Autodesk Fusion 360 part; units mm, degrees
(part 2 of 4)
sketch "Sketch2 (2)" plane through (0, 0, 6) normal (0, 0, 1) x (-1, 0, 0)
  arc A0 (-38.0356, 4.8944) -> (-38.1711, 3.692) centre (0, 0) ccw
  arc A1 (-39.2367, 2.7907) -> (-38.1711, 3.692) centre (-39.1664, 3.7883) ccw
  line L0 (-39.2367, 2.7907) -> (-39.3676, 2.8)
  spline S0 degree 5 poles (-39.3676, 2.8) (-39.3839, 2.8011) (-39.4163, 2.803) (-39.4649, 2.8047) (-39.5299, 2.8047) (-39.6111, 2.8017) (-39.6923, 2.7966) (-39.7736, 2.79) (-39.855, 2.7828) (-39.9363, 2.775) (-40.0176, 2.7667) (-40.099, 2.7577) (-40.1803, 2.7478) (-40.2616, 2.7369) (-40.343, 2.7249) (-40.4243, 2.7119) (-40.5056, 2.6981) (-40.5868, 2.6836) (-40.6681, 2.6685) (-40.7493, 2.6528) (-40.8305, 2.6365) (-40.9117, 2.6196) (-40.9928, 2.6021) (-41.074, 2.5839) (-41.1551, 2.5651) (-41.2361, 2.5457) (-41.3171, 2.5256) (-41.3981, 2.505) (-41.4791, 2.4839) (-41.56, 2.4622) (-41.6408, 2.44) (-41.7216, 2.4173) (-41.8024, 2.3941) (-41.8832, 2.3703) (-41.9638, 2.346) (-42.0445, 2.3213) (-42.1251, 2.296) (-42.2056, 2.2702) (-42.2861, 2.244) (-42.3666, 2.2173) (-42.447, 2.1901) (-42.5273, 2.1624) (-42.6076, 2.1343) (-42.6878, 2.1058) (-42.768, 2.0768) (-42.8481, 2.0473) (-42.9282, 2.0174) (-43.0082, 1.9871) (-43.0881, 1.9563) (-43.168, 1.9251) (-43.2479, 1.8935) (-43.3276, 1.8614) (-43.4073, 1.829) (-43.4869, 1.7961) (-43.5665, 1.7628) (-43.646, 1.7291) (-43.7254, 1.695) (-43.8048, 1.6605) (-43.8841, 1.6256) (-43.9633, 1.5903) (-44.0425, 1.5546) (-44.1216, 1.5185) (-44.2006, 1.482) (-44.2795, 1.4452) (-44.3584, 1.4079) (-44.4372, 1.3703) (-44.5159, 1.3323) (-44.5946, 1.2939) (-44.6732, 1.2552) (-44.7516, 1.2161) (-44.8301, 1.1766) (-44.8927, 1.1447) (-44.9397, 1.1206) (-44.971, 1.1045) (-44.9866, 1.0964) knots 0 0 0 0 0 0 0.01428571 0.02857143 0.04285714 0.05714286 0.07142857 0.08571429 0.1 0.11428571 0.12857143 0.14285714 0.15714286 0.17142857 0.18571429 0.2 0.21428571 0.22857143 0.24285714 0.25714286 0.27142857 0.28571429 0.3 0.31428571 0.32857143 0.34285714 0.35714286 0.37142857 0.38571429 0.4 0.41428571 0.42857143 0.44285714 0.45714286 0.47142857 0.48571429 0.5 0.51428571 0.52857143 0.54285714 0.55714286 0.57142857 0.58571429 0.6 0.61428571 0.62857143 0.64285714 0.65714286 0.67142857 0.68571429 0.7 0.71428571 0.72857143 0.74285714 0.75714286 0.77142857 0.78571429 0.8 0.81428571 0.82857143 0.84285714 0.85714286 0.87142857 0.88571429 0.9 0.91428571 0.92857143 0.94285714 0.95714286 0.97142857 0.98571429 1 1 1 1 1 1
  arc A2 (-44.9866, 1.0964) -> (-44.9866, -1.0964) centre (0, 0) ccw
  spline S1 degree 5 poles (-44.9866, -1.0964) (-44.971, -1.1045) (-44.9397, -1.1206) (-44.8927, -1.1447) (-44.8301, -1.1766) (-44.7516, -1.2161) (-44.6732, -1.2552) (-44.5946, -1.2939) (-44.5159, -1.3323) (-44.4372, -1.3703) (-44.3584, -1.4079) (-44.2795, -1.4452) (-44.2006, -1.482) (-44.1216, -1.5185) (-44.0425, -1.5546) (-43.9633, -1.5903) (-43.8841, -1.6256) (-43.8048, -1.6605) (-43.7254, -1.695) (-43.646, -1.7291) (-43.5665, -1.7628) (-43.4869, -1.7961) (-43.4073, -1.829) (-43.3276, -1.8614) (-43.2479, -1.8935) (-43.168, -1.9251) (-43.0881, -1.9563) (-43.0082, -1.9871) (-42.9282, -2.0174) (-42.8481, -2.0473) (-42.768, -2.0768) (-42.6878, -2.1058) (-42.6076, -2.1343) (-42.5273, -2.1624) (-42.447, -2.1901) (-42.3666, -2.2173) (-42.2861, -2.244) (-42.2056, -2.2702) (-42.1251, -2.296) (-42.0445, -2.3213) (-41.9638, -2.346) (-41.8832, -2.3703) (-41.8024, -2.3941) (-41.7216, -2.4173) (-41.6408, -2.44) (-41.56, -2.4622) (-41.4791, -2.4839) (-41.3981, -2.505) (-41.3171, -2.5256) (-41.2361, -2.5457) (-41.1551, -2.5651) (-41.074, -2.5839) (-40.9928, -2.6021) (-40.9117, -2.6196) (-40.8305, -2.6365) (-40.7493, -2.6528) (-40.6681, -2.6685) (-40.5868, -2.6836) (-40.5056, -2.6981) (-40.4243, -2.7119) (-40.343, -2.7249) (-40.2616, -2.7369) (-40.1803, -2.7478) (-40.099, -2.7577) (-40.0176, -2.7667) (-39.9363, -2.775) (-39.855, -2.7828) (-39.7736, -2.79) (-39.6923, -2.7966) (-39.6111, -2.8017) (-39.5299, -2.8047) (-39.4649, -2.8047) (-39.4163, -2.803) (-39.3839, -2.8011) (-39.3676, -2.8) knots -1 -1 -1 -1 -1 -1 -0.98571429 -0.97142857 -0.95714286 -0.94285714 -0.92857143 -0.91428571 -0.9 -0.88571429 -0.87142857 -0.85714286 -0.84285714 -0.82857143 -0.81428571 -0.8 -0.78571429 -0.77142857 -0.75714286 -0.74285714 -0.72857143 -0.71428571 -0.7 -0.68571429 -0.67142857 -0.65714286 -0.64285714 -0.62857143 -0.61428571 -0.6 -0.58571429 -0.57142857 -0.55714286 -0.54285714 -0.52857143 -0.51428571 -0.5 -0.48571429 -0.47142857 -0.45714286 -0.44285714 -0.42857143 -0.41428571 -0.4 -0.38571429 -0.37142857 -0.35714286 -0.34285714 -0.32857143 -0.31428571 -0.3 -0.28571429 -0.27142857 -0.25714286 -0.24285714 -0.22857143 -0.21428571 -0.2 -0.18571429 -0.17142857 -0.15714286 -0.14285714 -0.12857143 -0.11428571 -0.1 -0.08571429 -0.07142857 -0.05714286 -0.04285714 -0.02857143 -0.01428571 0 0 0 0 0 0
  line L1 (-39.3676, -2.8) -> (-39.2367, -2.7907)
  arc A3 (-38.1711, -3.692) -> (-39.2367, -2.7907) centre (-39.1664, -3.7883) ccw
  arc A4 (-38.1711, -3.692) -> (-38.0356, -4.8944) centre (0, 0) ccw
  arc A5 (-38.874, -6.0102) -> (-38.0356, -4.8944) centre (-39.0274, -5.0221) ccw
  line L2 (-38.874, -6.0102) -> (-39.0037, -6.0303)
  spline S2 degree 5 poles (-39.0037, -6.0303) (-39.0197, -6.0328) (-39.0518, -6.0382) (-39.0996, -6.0474) (-39.1629, -6.0618) (-39.2414, -6.0828) (-39.3195, -6.1059) (-39.3973, -6.1304) (-39.4749, -6.1556) (-39.5525, -6.1813) (-39.63, -6.2074) (-39.7073, -6.2343) (-39.7844, -6.262) (-39.8612, -6.2908) (-39.9378, -6.3206) (-40.0142, -6.3513) (-40.0904, -6.3829) (-40.1664, -6.4151) (-40.2422, -6.4479) (-40.3179, -6.4813) (-40.3935, -6.5152) (-40.4689, -6.5498) (-40.5441, -6.5849) (-40.6191, -6.6207) (-40.694, -6.6571) (-40.7687, -6.6941) (-40.8432, -6.7316) (-40.9176, -6.7697) (-40.9918, -6.8084) (-41.0659, -6.8475) (-41.1398, -6.8871) (-41.2135, -6.9272) (-41.2871, -6.9679) (-41.3605, -7.009) (-41.4338, -7.0506) (-41.5069, -7.0927) (-41.5798, -7.1353) (-41.6526, -7.1783) (-41.7253, -7.2218) (-41.7978, -7.2658) (-41.8701, -7.3102) (-41.9423, -7.355) (-42.0143, -7.4003) (-42.0861, -7.4459) (-42.1579, -7.4921) (-42.2294, -7.5386) (-42.3008, -7.5856) (-42.3721, -7.633) (-42.4432, -7.6808) (-42.5141, -7.7289) (-42.5849, -7.7775) (-42.6555, -7.8265) (-42.726, -7.8759) (-42.7963, -7.9257) (-42.8665, -7.9759) (-42.9365, -8.0264) (-43.0063, -8.0773) (-43.076, -8.1286) (-43.1456, -8.1803) (-43.215, -8.2323) (-43.2842, -8.2848) (-43.3533, -8.3375) (-43.4222, -8.3907) (-43.491, -8.4442) (-43.5596, -8.498) (-43.628, -8.5523) (-43.6963, -8.6068) (-43.7644, -8.6617) (-43.8324, -8.717) (-43.9002, -8.7726) (-43.9679, -8.8285) (-44.0219, -8.8736) (-44.0623, -8.9075) (-44.0893, -8.9302) (-44.1027, -8.9415) knots 0 0 0 0 0 0 0.01428571 0.02857143 0.04285714 0.05714286 0.07142857 0.08571429 0.1 0.11428571 0.12857143 0.14285714 0.15714286 0.17142857 0.18571429 0.2 0.21428571 0.22857143 0.24285714 0.25714286 0.27142857 0.28571429 0.3 0.31428571 0.32857143 0.34285714 0.35714286 0.37142857 0.38571429 0.4 0.41428571 0.42857143 0.44285714 0.45714286 0.47142857 0.48571429 0.5 0.51428571 0.52857143 0.54285714 0.55714286 0.57142857 0.58571429 0.6 0.61428571 0.62857143 0.64285714 0.65714286 0.67142857 0.68571429 0.7 0.71428571 0.72857143 0.74285714 0.75714286 0.77142857 0.78571429 0.8 0.81428571 0.82857143 0.84285714 0.85714286 0.87142857 0.88571429 0.9 0.91428571 0.92857143 0.94285714 0.95714286 0.97142857 0.98571429 1 1 1 1 1 1
  arc A6 (-44.1027, -8.9415) -> (-43.6148, -11.0794) centre (0, 0) ccw
  spline S3 degree 5 poles (-43.6148, -11.0794) (-43.5977, -11.0838) (-43.5636, -11.0926) (-43.5125, -11.1056) (-43.4443, -11.1227) (-43.359, -11.1438) (-43.2738, -11.1644) (-43.1886, -11.1847) (-43.1034, -11.2046) (-43.0182, -11.2242) (-42.933, -11.2433) (-42.8478, -11.2621) (-42.7626, -11.2804) (-42.6775, -11.2984) (-42.5923, -11.316) (-42.5072, -11.3332) (-42.4221, -11.35) (-42.337, -11.3664) (-42.252, -11.3823) (-42.167, -11.3979) (-42.0819, -11.4131) (-41.997, -11.4278) (-41.912, -11.4422) (-41.8271, -11.4561) (-41.7422, -11.4696) (-41.6573, -11.4826) (-41.5725, -11.4953) (-41.4877, -11.5075) (-41.403, -11.5193) (-41.3183, -11.5306) (-41.2336, -11.5415) (-41.149, -11.5519) (-41.0644, -11.5619) (-40.9799, -11.5715) (-40.8954, -11.5805) (-40.811, -11.5891) (-40.7266, -11.5973) (-40.6423, -11.6049) (-40.558, -11.6121) (-40.4738, -11.6188) (-40.3897, -11.6251) (-40.3056, -11.6308) (-40.2216, -11.636) (-40.1377, -11.6406) (-40.0538, -11.6448) (-39.9701, -11.6484) (-39.8864, -11.6516) (-39.8028, -11.6542) (-39.7192, -11.6562) (-39.6358, -11.6577) (-39.5524, -11.6587) (-39.4692, -11.659) (-39.3861, -11.6586) (-39.303, -11.6577) (-39.2201, -11.656) (-39.1373, -11.6538) (-39.0547, -11.6511) (-38.9721, -11.6477) (-38.8896, -11.6438) (-38.8073, -11.6392) (-38.7251, -11.6337) (-38.6432, -11.6273) (-38.5615, -11.6199) (-38.48, -11.6114) (-38.3987, -11.6021) (-38.3175, -11.5921) (-38.2365, -11.5816) (-38.1556, -11.5706) (-38.0749, -11.5588) (-37.9945, -11.5458) (-37.9147, -11.5306) (-37.8514, -11.5162) (-37.8043, -11.5037) (-37.7731, -11.4946) (-37.7576, -11.4899) knots -1 -1 -1 -1 -1 -1 -0.98571429 -0.97142857 -0.95714286 -0.94285714 -0.92857143 -0.91428571 -0.9 -0.88571429 -0.87142857 -0.85714286 -0.84285714 -0.82857143 -0.81428571 -0.8 -0.78571429 -0.77142857 -0.75714286 -0.74285714 -0.72857143 -0.71428571 -0.7 -0.68571429 -0.67142857 -0.65714286 -0.64285714 -0.62857143 -0.61428571 -0.6 -0.58571429 -0.57142857 -0.55714286 -0.54285714 -0.52857143 -0.51428571 -0.5 -0.48571429 -0.47142857 -0.45714286 -0.44285714 -0.42857143 -0.41428571 -0.4 -0.38571429 -0.37142857 -0.35714286 -0.34285714 -0.32857143 -0.31428571 -0.3 -0.28571429 -0.27142857 -0.25714286 -0.24285714 -0.22857143 -0.21428571 -0.2 -0.18571429 -0.17142857 -0.15714286 -0.14285714 -0.12857143 -0.11428571 -0.1 -0.08571429 -0.07142857 -0.05714286 -0.04285714 -0.02857143 -0.01428571 0 0 0 0 0 0
  line L3 (-37.7576, -11.4899) -> (-37.632, -11.4518)
  arc A7 (-36.3925, -12.0933) -> (-37.632, -11.4518) centre (-37.3415, -12.4086) ccw
  arc A8 (-36.3925, -12.0933) -> (-35.9928, -13.2354) centre (0, 0) ccw
  arc A9 (-36.5619, -14.5098) -> (-35.9928, -13.2354) centre (-36.9314, -13.5806) ccw
  line L4 (-36.5619, -14.5098) -> (-36.6839, -14.5583)
  spline S4 degree 5 poles (-36.6839, -14.5583) (-36.699, -14.5643) (-36.729, -14.5767) (-36.7736, -14.5962) (-36.8321, -14.6244) (-36.904, -14.6623) (-36.975, -14.7022) (-37.0454, -14.7434) (-37.1155, -14.7852) (-37.1854, -14.8275) (-37.2551, -14.8703) (-37.3245, -14.9137) (-37.3935, -14.9579) (-37.462, -15.003) (-37.5301, -15.0491) (-37.5977, -15.0961) (-37.6649, -15.1438) (-37.7319, -15.1921) (-37.7985, -15.241) (-37.8649, -15.2904) (-37.931, -15.3403) (-37.9968, -15.3907) (-38.0623, -15.4417) (-38.1275, -15.4933) (-38.1924, -15.5454) (-38.257, -15.5981) (-38.3213, -15.6513) (-38.3853, -15.705) (-38.449, -15.7592) (-38.5125, -15.8138) (-38.5758, -15.8689) (-38.6387, -15.9244) (-38.7014, -15.9804) (-38.7639, -16.0368) (-38.826, -16.0937) (-38.8879, -16.151) (-38.9496, -16.2088) (-39.011, -16.2669) (-39.0721, -16.3255) (-39.133, -16.3845) (-39.1937, -16.4438) (-39.254, -16.5036) (-39.3142, -16.5638) (-39.3741, -16.6243) (-39.4337, -16.6852) (-39.4931, -16.7465) (-39.5523, -16.8082) (-39.6112, -16.8703) (-39.6699, -16.9327) (-39.7283, -16.9954) (-39.7865, -17.0586) (-39.8445, -17.122) (-39.9022, -17.1859) (-39.9597, -17.25) (-40.0169, -17.3146) (-40.0739, -17.3794) (-40.1307, -17.4446) (-40.1872, -17.5101) (-40.2435, -17.576) (-40.2996, -17.6422) (-40.3554, -17.7087) (-40.411, -17.7755) (-40.4664, -17.8427) (-40.5215, -17.9101) (-40.5764, -17.9779) (-40.6311, -18.046) (-40.6855, -18.1144) (-40.7398, -18.1831) (-40.7937, -18.2521) (-40.8475, -18.3214) (-40.901, -18.391) (-40.9436, -18.4469) (-40.9755, -18.4889) (-40.9967, -18.5171) (-41.0073, -18.5311) knots 0 0 0 0 0 0 0.01428571 0.02857143 0.04285714 0.05714286 0.07142857 0.08571429 0.1 0.11428571 0.12857143 0.14285714 0.15714286 0.17142857 0.18571429 0.2 0.21428571 0.22857143 0.24285714 0.25714286 0.27142857 0.28571429 0.3 0.31428571 0.32857143 0.34285714 0.35714286 0.37142857 0.38571429 0.4 0.41428571 0.42857143 0.44285714 0.45714286 0.47142857 0.48571429 0.5 0.51428571 0.52857143 0.54285714 0.55714286 0.57142857 0.58571429 0.6 0.61428571 0.62857143 0.64285714 0.65714286 0.67142857 0.68571429 0.7 0.71428571 0.72857143 0.74285714 0.75714286 0.77142857 0.78571429 0.8 0.81428571 0.82857143 0.84285714 0.85714286 0.87142857 0.88571429 0.9 0.91428571 0.92857143 0.94285714 0.95714286 0.97142857 0.98571429 1 1 1 1 1 1
  arc A10 (-41.0073, -18.5311) -> (-40.0558, -20.5068) centre (0, 0) ccw
  spline S5 degree 5 poles (-40.0558, -20.5068) (-40.0382, -20.5073) (-40.003, -20.5083) (-39.9503, -20.5096) (-39.88, -20.5111) (-39.7922, -20.5127) (-39.7045, -20.5138) (-39.6169, -20.5147) (-39.5294, -20.5151) (-39.442, -20.5152) (-39.3547, -20.5149) (-39.2675, -20.5142) (-39.1803, -20.5132) (-39.0933, -20.5118) (-39.0064, -20.51) (-38.9196, -20.5078) (-38.8329, -20.5052) (-38.7463, -20.5023) (-38.6598, -20.4989) (-38.5735, -20.4952) (-38.4872, -20.491) (-38.4011, -20.4865) (-38.3151, -20.4816) (-38.2292, -20.4762) (-38.1434, -20.4705) (-38.0578, -20.4644) (-37.9723, -20.4578) (-37.8869, -20.4509) (-37.8016, -20.4435) (-37.7165, -20.4357) (-37.6316, -20.4275) (-37.5467, -20.4188) (-37.4621, -20.4097) (-37.3775, -20.4002) (-37.2932, -20.3903) (-37.2089, -20.3799) (-37.1249, -20.369) (-37.041, -20.3577) (-36.9572, -20.346) (-36.8736, -20.3338) (-36.7902, -20.3211) (-36.707, -20.308) (-36.6239, -20.2944) (-36.5411, -20.2803) (-36.4584, -20.2657) (-36.3759, -20.2506) (-36.2936, -20.235) (-36.2115, -20.2189) (-36.1296, -20.2023) (-36.0479, -20.1852) (-35.9665, -20.1676) (-35.8852, -20.1494) (-35.8043, -20.1305) (-35.7236, -20.1111) (-35.6431, -20.0911) (-35.5629, -20.0705) (-35.4829, -20.0494) (-35.4031, -20.0278) (-35.3236, -20.0056) (-35.2443, -19.9828) (-35.1655, -19.9592) (-35.087, -19.9347) (-35.009, -19.9093) (-34.9314, -19.8829) (-34.8542, -19.8557) (-34.7773, -19.8279) (-34.7007, -19.7996) (-34.6243, -19.7709) (-34.5482, -19.7415) (-34.4727, -19.7109) (-34.3983, -19.6783) (-34.3398, -19.6501) (-34.2967, -19.6275) (-34.2683, -19.6117) (-34.2542, -19.6037) knots -1 -1 -1 -1 -1 -1 -0.98571429 -0.97142857 -0.95714286 -0.94285714 -0.92857143 -0.91428571 -0.9 -0.88571429 -0.87142857 -0.85714286 -0.84285714 -0.82857143 -0.81428571 -0.8 -0.78571429 -0.77142857 -0.75714286 -0.74285714 -0.72857143 -0.71428571 -0.7 -0.68571429 -0.67142857 -0.65714286 -0.64285714 -0.62857143 -0.61428571 -0.6 -0.58571429 -0.57142857 -0.55714286 -0.54285714 -0.52857143 -0.51428571 -0.5 -0.48571429 -0.47142857 -0.45714286 -0.44285714 -0.42857143 -0.41428571 -0.4 -0.38571429 -0.37142857 -0.35714286 -0.34285714 -0.32857143 -0.31428571 -0.3 -0.28571429 -0.27142857 -0.25714286 -0.24285714 -0.22857143 -0.21428571 -0.2 -0.18571429 -0.17142857 -0.15714286 -0.14285714 -0.12857143 -0.11428571 -0.1 -0.08571429 -0.07142857 -0.05714286 -0.04285714 -0.02857143 -0.01428571 0 0 0 0 0 0
  line L5 (-34.2542, -19.6037) -> (-34.1402, -19.5386)
  arc A11 (-32.789, -19.8882) -> (-34.1402, -19.5386) centre (-33.6441, -20.4068) ccw
  arc A12 (-32.789, -19.8882) -> (-32.1453, -20.9127) centre (0, 0) ccw
  arc A13 (-32.4165, -22.2818) -> (-32.1453, -20.9127) centre (-32.9835, -21.4581) ccw
  line L6 (-32.4165, -22.2818) -> (-32.5246, -22.3562)
  spline S6 degree 5 poles (-32.5246, -22.3562) (-32.538, -22.3654) (-32.5645, -22.3842) (-32.6036, -22.4132) (-32.6544, -22.4536) (-32.7161, -22.5066) (-32.7764, -22.5613) (-32.8358, -22.6171) (-32.8949, -22.6735) (-32.9536, -22.7303) (-33.012, -22.7875) (-33.07, -22.8452) (-33.1275, -22.9037) (-33.1843, -22.9629) (-33.2404, -23.023) (-33.2958, -23.0838) (-33.3508, -23.1453) (-33.4053, -23.2074) (-33.4594, -23.2698) (-33.5131, -23.3328) (-33.5664, -23.3961) (-33.6194, -23.4599) (-33.6719, -23.5242) (-33.724, -23.589) (-33.7756, -23.6543) (-33.8269, -23.72) (-33.8777, -23.7862) (-33.9282, -23.8528) (-33.9783, -23.9198) (-34.028, -23.9872) (-34.0774, -24.0549) (-34.1265, -24.1231) (-34.1751, -24.1916) (-34.2234, -24.2605) (-34.2714, -24.3298) (-34.319, -24.3995) (-34.3662, -24.4695) (-34.4132, -24.5399) (-34.4597, -24.6106) (-34.506, -24.6816) (-34.5519, -24.753) (-34.5975, -24.8247) (-34.6427, -24.8967) (-34.6876, -24.9691) (-34.7322, -25.0417) (-34.7765, -25.1147) (-34.8205, -25.188) (-34.8641, -25.2616) (-34.9074, -25.3355) (-34.9504, -25.4097) (-34.9931, -25.4842) (-35.0355, -25.559) (-35.0775, -25.6341) (-35.1193, -25.7094) (-35.1608, -25.7851) (-35.2019, -25.861) (-35.2427, -25.9372) (-35.2833, -26.0136) (-35.3235, -26.0904) (-35.3635, -26.1674) (-35.4031, -26.2446) (-35.4424, -26.3221) (-35.4815, -26.3999) (-35.5202, -26.478) (-35.5586, -26.5563) (-35.5968, -26.6348) (-35.6346, -26.7136) (-35.6722, -26.7926) (-35.7095, -26.8719) (-35.7465, -26.9514) (-35.7831, -27.0312) (-35.8123, -27.0952) (-35.834, -27.1433) (-35.8484, -27.1754) (-35.8556, -27.1915) knots 0 0 0 0 0 0 0.01428571 0.02857143 0.04285714 0.05714286 0.07142857 0.08571429 0.1 0.11428571 0.12857143 0.14285714 0.15714286 0.17142857 0.18571429 0.2 0.21428571 0.22857143 0.24285714 0.25714286 0.27142857 0.28571429 0.3 0.31428571 0.32857143 0.34285714 0.35714286 0.37142857 0.38571429 0.4 0.41428571 0.42857143 0.44285714 0.45714286 0.47142857 0.48571429 0.5 0.51428571 0.52857143 0.54285714 0.55714286 0.57142857 0.58571429 0.6 0.61428571 0.62857143 0.64285714 0.65714286 0.67142857 0.68571429 0.7 0.71428571 0.72857143 0.74285714 0.75714286 0.77142857 0.78571429 0.8 0.81428571 0.82857143 0.84285714 0.85714286 0.87142857 0.88571429 0.9 0.91428571 0.92857143 0.94285714 0.95714286 0.97142857 0.98571429 1 1 1 1 1 1
  arc A14 (-35.8556, -27.1915) -> (-34.4884, -28.9059) centre (0, 0) ccw
  spline S7 degree 5 poles (-34.4884, -28.9059) (-34.4711, -28.9025) (-34.4366, -28.8956) (-34.3848, -28.8851) (-34.316, -28.871) (-34.23, -28.853) (-34.1443, -28.8346) (-34.0587, -28.8159) (-33.9733, -28.7969) (-33.888, -28.7775) (-33.803, -28.7578) (-33.7181, -28.7377) (-33.6334, -28.7173) (-33.5489, -28.6966) (-33.4645, -28.6755) (-33.3804, -28.654) (-33.2964, -28.6322) (-33.2127, -28.6101) (-33.1291, -28.5876) (-33.0457, -28.5647) (-32.9626, -28.5415) (-32.8796, -28.5179) (-32.7969, -28.494) (-32.7143, -28.4697) (-32.632, -28.445) (-32.5498, -28.4199) (-32.4679, -28.3945) (-32.3862, -28.3687) (-32.3048, -28.3426) (-32.2235, -28.316) (-32.1425, -28.2891) (-32.0618, -28.2618) (-31.9812, -28.2341) (-31.9009, -28.206) (-31.8209, -28.1775) (-31.7411, -28.1487) (-31.6615, -28.1194) (-31.5822, -28.0897) (-31.5032, -28.0596) (-31.4244, -28.0291) (-31.3459, -27.9982) (-31.2677, -27.9669) (-31.1898, -27.9351) (-31.1121, -27.9029) (-31.0348, -27.8703) (-30.9577, -27.8372) (-30.881, -27.8037) (-30.8045, -27.7698) (-30.7283, -27.7354) (-30.6525, -27.7006) (-30.577, -27.6652) (-30.5019, -27.6294) (-30.4271, -27.593) (-30.3527, -27.5561) (-30.2788, -27.5187) (-30.2051, -27.4808) (-30.1318, -27.4424) (-30.0589, -27.4036) (-29.9863, -27.3643) (-29.9141, -27.3244) (-29.8425, -27.2838) (-29.7714, -27.2425) (-29.701, -27.2004) (-29.6312, -27.1574) (-29.562, -27.1137) (-29.4933, -27.0694) (-29.4248, -27.0248) (-29.3567, -26.9798) (-29.2891, -26.9342) (-29.2223, -26.8876) (-29.157, -26.8393) (-29.1062, -26.7988) (-29.0692, -26.7671) (-29.0451, -26.7454) (-29.0331, -26.7344) knots -1 -1 -1 -1 -1 -1 -0.98571429 -0.97142857 -0.95714286 -0.94285714 -0.92857143 -0.91428571 -0.9 -0.88571429 -0.87142857 -0.85714286 -0.84285714 -0.82857143 -0.81428571 -0.8 -0.78571429 -0.77142857 -0.75714286 -0.74285714 -0.72857143 -0.71428571 -0.7 -0.68571429 -0.67142857 -0.65714286 -0.64285714 -0.62857143 -0.61428571 -0.6 -0.58571429 -0.57142857 -0.55714286 -0.54285714 -0.52857143 -0.51428571 -0.5 -0.48571429 -0.47142857 -0.45714286 -0.44285714 -0.42857143 -0.41428571 -0.4 -0.38571429 -0.37142857 -0.35714286 -0.34285714 -0.32857143 -0.31428571 -0.3 -0.28571429 -0.27142857 -0.25714286 -0.24285714 -0.22857143 -0.21428571 -0.2 -0.18571429 -0.17142857 -0.15714286 -0.14285714 -0.12857143 -0.11428571 -0.1 -0.08571429 -0.07142857 -0.05714286 -0.04285714 -0.02857143 -0.01428571 0 0 0 0 0 0
  line L7 (-29.0331, -26.7344) -> (-28.9365, -26.6456)
  arc A15 (-27.5414, -26.6858) -> (-28.9365, -26.6456) centre (-28.2596, -27.3817) ccw
  arc A16 (-27.5414, -26.6858) -> (-26.6858, -27.5414) centre (0, 0) ccw
  arc A17 (-26.6456, -28.9365) -> (-26.6858, -27.5414) centre (-27.3817, -28.2596) ccw
  line L8 (-26.6456, -28.9365) -> (-26.7344, -29.0331)
  spline S8 degree 5 poles (-26.7344, -29.0331) (-26.7454, -29.0451) (-26.7671, -29.0692) (-26.7988, -29.1062) (-26.8393, -29.157) (-26.8876, -29.2223) (-26.9342, -29.2891) (-26.9798, -29.3567) (-27.0248, -29.4248) (-27.0694, -29.4933) (-27.1137, -29.562) (-27.1574, -29.6312) (-27.2004, -29.701) (-27.2425, -29.7714) (-27.2838, -29.8425) (-27.3244, -29.9141) (-27.3643, -29.9863) (-27.4036, -30.0589) (-27.4424, -30.1318) (-27.4808, -30.2051) (-27.5187, -30.2788) (-27.5561, -30.3527) (-27.593, -30.4271) (-27.6294, -30.5019) (-27.6652, -30.577) (-27.7006, -30.6525) (-27.7354, -30.7283) (-27.7698, -30.8045) (-27.8037, -30.881) (-27.8372, -30.9577) (-27.8703, -31.0348) (-27.9029, -31.1121) (-27.9351, -31.1898) (-27.9669, -31.2677) (-27.9982, -31.3459) (-28.0291, -31.4244) (-28.0596, -31.5032) (-28.0897, -31.5822) (-28.1194, -31.6615) (-28.1487, -31.7411) (-28.1775, -31.8209) (-28.206, -31.9009) (-28.2341, -31.9812) (-28.2618, -32.0618) (-28.2891, -32.1425) (-28.316, -32.2235) (-28.3426, -32.3048) (-28.3687, -32.3862) (-28.3945, -32.4679) (-28.4199, -32.5498) (-28.445, -32.632) (-28.4697, -32.7143) (-28.494, -32.7969) (-28.5179, -32.8796) (-28.5415, -32.9626) (-28.5647, -33.0457) (-28.5876, -33.1291) (-28.6101, -33.2127) (-28.6322, -33.2964) (-28.654, -33.3804) (-28.6755, -33.4645) (-28.6966, -33.5489) (-28.7173, -33.6334) (-28.7377, -33.7181) (-28.7578, -33.803) (-28.7775, -33.888) (-28.7969, -33.9733) (-28.8159, -34.0587) (-28.8346, -34.1443) (-28.853, -34.23) (-28.871, -34.316) (-28.8851, -34.3848) (-28.8956, -34.4366) (-28.9025, -34.4711) (-28.9059, -34.4884) knots 0 0 0 0 0 0 0.01428571 0.02857143 0.04285714 0.05714286 0.07142857 0.08571429 0.1 0.11428571 0.12857143 0.14285714 0.15714286 0.17142857 0.18571429 0.2 0.21428571 0.22857143 0.24285714 0.25714286 0.27142857 0.28571429 0.3 0.31428571 0.32857143 0.34285714 0.35714286 0.37142857 0.38571429 0.4 0.41428571 0.42857143 0.44285714 0.45714286 0.47142857 0.48571429 0.5 0.51428571 0.52857143 0.54285714 0.55714286 0.57142857 0.58571429 0.6 0.61428571 0.62857143 0.64285714 0.65714286 0.67142857 0.68571429 0.7 0.71428571 0.72857143 0.74285714 0.75714286 0.77142857 0.78571429 0.8 0.81428571 0.82857143 0.84285714 0.85714286 0.87142857 0.88571429 0.9 0.91428571 0.92857143 0.94285714 0.95714286 0.97142857 0.98571429 1 1 1 1 1 1
  arc A18 (-28.9059, -34.4884) -> (-27.1915, -35.8556) centre (0, 0) ccw
  spline S9 degree 5 poles (-27.1915, -35.8556) (-27.1754, -35.8484) (-27.1433, -35.834) (-27.0952, -35.8123) (-27.0312, -35.7831) (-26.9514, -35.7465) (-26.8719, -35.7095) (-26.7926, -35.6722) (-26.7136, -35.6346) (-26.6348, -35.5968) (-26.5563, -35.5586) (-26.478, -35.5202) (-26.3999, -35.4815) (-26.3221, -35.4424) (-26.2446, -35.4031) (-26.1674, -35.3635) (-26.0904, -35.3235) (-26.0136, -35.2833) (-25.9372, -35.2427) (-25.861, -35.2019) (-25.7851, -35.1608) (-25.7094, -35.1193) (-25.6341, -35.0775) (-25.559, -35.0355) (-25.4842, -34.9931) (-25.4097, -34.9504) (-25.3355, -34.9074) (-25.2616, -34.8641) (-25.188, -34.8205) (-25.1147, -34.7765) (-25.0417, -34.7322) (-24.9691, -34.6876) (-24.8967, -34.6427) (-24.8247, -34.5975) (-24.753, -34.5519) (-24.6816, -34.506) (-24.6106, -34.4597) (-24.5399, -34.4132) (-24.4695, -34.3662) (-24.3995, -34.319) (-24.3298, -34.2714) (-24.2605, -34.2234) (-24.1916, -34.1751) (-24.1231, -34.1265) (-24.0549, -34.0774) (-23.9872, -34.028) (-23.9198, -33.9783) (-23.8528, -33.9282) (-23.7862, -33.8777) (-23.72, -33.8269) (-23.6543, -33.7756) (-23.589, -33.724) (-23.5242, -33.6719) (-23.4599, -33.6194) (-23.3961, -33.5664) (-23.3328, -33.5131) (-23.2698, -33.4594) (-23.2074, -33.4053) (-23.1453, -33.3508) (-23.0838, -33.2958) (-23.023, -33.2404) (-22.9629, -33.1843) (-22.9037, -33.1275) (-22.8452, -33.07) (-22.7875, -33.012) (-22.7303, -32.9536) (-22.6735, -32.8949) (-22.6171, -32.8358) (-22.5613, -32.7764) (-22.5066, -32.7161) (-22.4536, -32.6544) (-22.4132, -32.6036) (-22.3842, -32.5645) (-22.3654, -32.538) (-22.3562, -32.5246) knots -1 -1 -1 -1 -1 -1 -0.98571429 -0.97142857 -0.95714286 -0.94285714 -0.92857143 -0.91428571 -0.9 -0.88571429 -0.87142857 -0.85714286 -0.84285714 -0.82857143 -0.81428571 -0.8 -0.78571429 -0.77142857 -0.75714286 -0.74285714 -0.72857143 -0.71428571 -0.7 -0.68571429 -0.67142857 -0.65714286 -0.64285714 -0.62857143 -0.61428571 -0.6 -0.58571429 -0.57142857 -0.55714286 -0.54285714 -0.52857143 -0.51428571 -0.5 -0.48571429 -0.47142857 -0.45714286 -0.44285714 -0.42857143 -0.41428571 -0.4 -0.38571429 -0.37142857 -0.35714286 -0.34285714 -0.32857143 -0.31428571 -0.3 -0.28571429 -0.27142857 -0.25714286 -0.24285714 -0.22857143 -0.21428571 -0.2 -0.18571429 -0.17142857 -0.15714286 -0.14285714 -0.12857143 -0.11428571 -0.1 -0.08571429 -0.07142857 -0.05714286 -0.04285714 -0.02857143 -0.01428571 0 0 0 0 0 0
  line L9 (-22.3562, -32.5246) -> (-22.2818, -32.4165)
  arc A19 (-20.9127, -32.1453) -> (-22.2818, -32.4165) centre (-21.4581, -32.9835) ccw
  arc A20 (-20.9127, -32.1453) -> (-19.8882, -32.789) centre (0, 0) ccw
  arc A21 (-19.5386, -34.1402) -> (-19.8882, -32.789) centre (-20.4068, -33.6441) ccw
  line L10 (-19.5386, -34.1402) -> (-19.6037, -34.2542)
  spline S10 degree 5 poles (-19.6037, -34.2542) (-19.6117, -34.2683) (-19.6275, -34.2967) (-19.6501, -34.3398) (-19.6783, -34.3983) (-19.7109, -34.4727) (-19.7415, -34.5482) (-19.7709, -34.6243) (-19.7996, -34.7007) (-19.8279, -34.7773) (-19.8557, -34.8542) (-19.8829, -34.9314) (-19.9093, -35.009) (-19.9347, -35.087) (-19.9592, -35.1655) (-19.9828, -35.2443) (-20.0056, -35.3236) (-20.0278, -35.4031) (-20.0494, -35.4829) (-20.0705, -35.5629) (-20.0911, -35.6431) (-20.1111, -35.7236) (-20.1305, -35.8043) (-20.1494, -35.8852) (-20.1676, -35.9665) (-20.1852, -36.0479) (-20.2023, -36.1296) (-20.2189, -36.2115) (-20.235, -36.2936) (-20.2506, -36.3759) (-20.2657, -36.4584) (-20.2803, -36.5411) (-20.2944, -36.6239) (-20.308, -36.707) (-20.3211, -36.7902) (-20.3338, -36.8736) (-20.346, -36.9572) (-20.3577, -37.041) (-20.369, -37.1249) (-20.3799, -37.2089) (-20.3903, -37.2932) (-20.4002, -37.3775) (-20.4097, -37.4621) (-20.4188, -37.5467) (-20.4275, -37.6316) (-20.4357, -37.7165) (-20.4435, -37.8016) (-20.4509, -37.8869) (-20.4578, -37.9723) (-20.4644, -38.0578) (-20.4705, -38.1434) (-20.4762, -38.2292) (-20.4816, -38.3151) (-20.4865, -38.4011) (-20.491, -38.4872) (-20.4952, -38.5735) (-20.4989, -38.6598) (-20.5023, -38.7463) (-20.5052, -38.8329) (-20.5078, -38.9196) (-20.51, -39.0064) (-20.5118, -39.0933) (-20.5132, -39.1803) (-20.5142, -39.2675) (-20.5149, -39.3547) (-20.5152, -39.442) (-20.5151, -39.5294) (-20.5147, -39.6169) (-20.5138, -39.7045) (-20.5127, -39.7922) (-20.5111, -39.88) (-20.5096, -39.9503) (-20.5083, -40.003) (-20.5073, -40.0382) (-20.5068, -40.0558) knots 0 0 0 0 0 0 0.01428571 0.02857143 0.04285714 0.05714286 0.07142857 0.08571429 0.1 0.11428571 0.12857143 0.14285714 0.15714286 0.17142857 0.18571429 0.2 0.21428571 0.22857143 0.24285714 0.25714286 0.27142857 0.28571429 0.3 0.31428571 0.32857143 0.34285714 0.35714286 0.37142857 0.38571429 0.4 0.41428571 0.42857143 0.44285714 0.45714286 0.47142857 0.48571429 0.5 0.51428571 0.52857143 0.54285714 0.55714286 0.57142857 0.58571429 0.6 0.61428571 0.62857143 0.64285714 0.65714286 0.67142857 0.68571429 0.7 0.71428571 0.72857143 0.74285714 0.75714286 0.77142857 0.78571429 0.8 0.81428571 0.82857143 0.84285714 0.85714286 0.87142857 0.88571429 0.9 0.91428571 0.92857143 0.94285714 0.95714286 0.97142857 0.98571429 1 1 1 1 1 1
  arc A22 (-20.5068, -40.0558) -> (-18.5311, -41.0073) centre (0, 0) ccw
  spline S11 degree 5 poles (-18.5311, -41.0073) (-18.5171, -40.9967) (-18.4889, -40.9755) (-18.4469, -40.9436) (-18.391, -40.901) (-18.3214, -40.8475) (-18.2521, -40.7937) (-18.1831, -40.7398) (-18.1144, -40.6855) (-18.046, -40.6311) (-17.9779, -40.5764) (-17.9101, -40.5215) (-17.8427, -40.4664) (-17.7755, -40.411) (-17.7087, -40.3554) (-17.6422, -40.2996) (-17.576, -40.2435) (-17.5101, -40.1872) (-17.4446, -40.1307) (-17.3794, -40.0739) (-17.3146, -40.0169) (-17.25, -39.9597) (-17.1859, -39.9022) (-17.122, -39.8445) (-17.0586, -39.7865) (-16.9954, -39.7283) (-16.9327, -39.6699) (-16.8703, -39.6112) (-16.8082, -39.5523) (-16.7465, -39.4931) (-16.6852, -39.4337) (-16.6243, -39.3741) (-16.5638, -39.3142) (-16.5036, -39.254) (-16.4438, -39.1937) (-16.3845, -39.133) (-16.3255, -39.0721) (-16.2669, -39.011) (-16.2088, -38.9496) (-16.151, -38.8879) (-16.0937, -38.826) (-16.0368, -38.7639) (-15.9804, -38.7014) (-15.9244, -38.6387) (-15.8689, -38.5758) (-15.8138, -38.5125) (-15.7592, -38.449) (-15.705, -38.3853) (-15.6513, -38.3213) (-15.5981, -38.257) (-15.5454, -38.1924) (-15.4933, -38.1275) (-15.4417, -38.0623) (-15.3907, -37.9968) (-15.3403, -37.931) (-15.2904, -37.8649) (-15.241, -37.7985) (-15.1921, -37.7319) (-15.1438, -37.6649) (-15.0961, -37.5977) (-15.0491, -37.5301) (-15.003, -37.462) (-14.9579, -37.3935) (-14.9137, -37.3245) (-14.8703, -37.2551) (-14.8275, -37.1854) (-14.7852, -37.1155) (-14.7434, -37.0454) (-14.7022, -36.975) (-14.6623, -36.904) (-14.6244, -36.8321) (-14.5962, -36.7736) (-14.5767, -36.729) (-14.5643, -36.699) (-14.5583, -36.6839) knots -1 -1 -1 -1 -1 -1 -0.98571429 -0.97142857 -0.95714286 -0.94285714 -0.92857143 -0.91428571 -0.9 -0.88571429 -0.87142857 -0.85714286 -0.84285714 -0.82857143 -0.81428571 -0.8 -0.78571429 -0.77142857 -0.75714286 -0.74285714 -0.72857143 -0.71428571 -0.7 -0.68571429 -0.67142857 -0.65714286 -0.64285714 -0.62857143 -0.61428571 -0.6 -0.58571429 -0.57142857 -0.55714286 -0.54285714 -0.52857143 -0.51428571 -0.5 -0.48571429 -0.47142857 -0.45714286 -0.44285714 -0.42857143 -0.41428571 -0.4 -0.38571429 -0.37142857 -0.35714286 -0.34285714 -0.32857143 -0.31428571 -0.3 -0.28571429 -0.27142857 -0.25714286 -0.24285714 -0.22857143 -0.21428571 -0.2 -0.18571429 -0.17142857 -0.15714286 -0.14285714 -0.12857143 -0.11428571 -0.1 -0.08571429 -0.07142857 -0.05714286 -0.04285714 -0.02857143 -0.01428571 0 0 0 0 0 0
  line L11 (-14.5583, -36.6839) -> (-14.5098, -36.5619)
  arc A23 (-13.2354, -35.9928) -> (-14.5098, -36.5619) centre (-13.5806, -36.9314) ccw
  arc A24 (-13.2354, -35.9928) -> (-12.0933, -36.3925) centre (0, 0) ccw
  arc A25 (-11.4518, -37.632) -> (-12.0933, -36.3925) centre (-12.4086, -37.3415) ccw
  line L12 (-11.4518, -37.632) -> (-11.4899, -37.7576)
  spline S12 degree 5 poles (-11.4899, -37.7576) (-11.4946, -37.7731) (-11.5037, -37.8043) (-11.5162, -37.8514) (-11.5306, -37.9147) (-11.5458, -37.9945) (-11.5588, -38.0749) (-11.5706, -38.1556) (-11.5816, -38.2365) (-11.5921, -38.3175) (-11.6021, -38.3987) (-11.6114, -38.48) (-11.6199, -38.5615) (-11.6273, -38.6432) (-11.6337, -38.7251) (-11.6392, -38.8073) (-11.6438, -38.8896) (-11.6477, -38.9721) (-11.6511, -39.0547) (-11.6538, -39.1373) (-11.656, -39.2201) (-11.6577, -39.303) (-11.6586, -39.3861) (-11.659, -39.4692) (-11.6587, -39.5524) (-11.6577, -39.6358) (-11.6562, -39.7192) (-11.6542, -39.8028) (-11.6516, -39.8864) (-11.6484, -39.9701) (-11.6448, -40.0538) (-11.6406, -40.1377) (-11.636, -40.2216) (-11.6308, -40.3056) (-11.6251, -40.3897) (-11.6188, -40.4738) (-11.6121, -40.558) (-11.6049, -40.6423) (-11.5973, -40.7266) (-11.5891, -40.811) (-11.5805, -40.8954) (-11.5715, -40.9799) (-11.5619, -41.0644) (-11.5519, -41.149) (-11.5415, -41.2336) (-11.5306, -41.3183) (-11.5193, -41.403) (-11.5075, -41.4877) (-11.4953, -41.5725) (-11.4826, -41.6573) (-11.4696, -41.7422) (-11.4561, -41.8271) (-11.4422, -41.912) (-11.4278, -41.997) (-11.4131, -42.0819) (-11.3979, -42.167) (-11.3823, -42.252) (-11.3664, -42.337) (-11.35, -42.4221) (-11.3332, -42.5072) (-11.316, -42.5923) (-11.2984, -42.6775) (-11.2804, -42.7626) (-11.2621, -42.8478) (-11.2433, -42.933) (-11.2242, -43.0182) (-11.2046, -43.1034) (-11.1847, -43.1886) (-11.1644, -43.2738) (-11.1438, -43.359) (-11.1227, -43.4443) (-11.1056, -43.5125) (-11.0926, -43.5636) (-11.0838, -43.5977) (-11.0794, -43.6148) knots 0 0 0 0 0 0 0.01428571 0.02857143 0.04285714 0.05714286 0.07142857 0.08571429 0.1 0.11428571 0.12857143 0.14285714 0.15714286 0.17142857 0.18571429 0.2 0.21428571 0.22857143 0.24285714 0.25714286 0.27142857 0.28571429 0.3 0.31428571 0.32857143 0.34285714 0.35714286 0.37142857 0.38571429 0.4 0.41428571 0.42857143 0.44285714 0.45714286 0.47142857 0.48571429 0.5 0.51428571 0.52857143 0.54285714 0.55714286 0.57142857 0.58571429 0.6 0.61428571 0.62857143 0.64285714 0.65714286 0.67142857 0.68571429 0.7 0.71428571 0.72857143 0.74285714 0.75714286 0.77142857 0.78571429 0.8 0.81428571 0.82857143 0.84285714 0.85714286 0.87142857 0.88571429 0.9 0.91428571 0.92857143 0.94285714 0.95714286 0.97142857 0.98571429 1 1 1 1 1 1
  arc A26 (-11.0794, -43.6148) -> (-8.9415, -44.1027) centre (0, 0) ccw
  spline S13 degree 5 poles (-8.9415, -44.1027) (-8.9302, -44.0893) (-8.9075, -44.0623) (-8.8736, -44.0219) (-8.8285, -43.9679) (-8.7726, -43.9002) (-8.717, -43.8324) (-8.6617, -43.7644) (-8.6068, -43.6963) (-8.5523, -43.628) (-8.498, -43.5596) (-8.4442, -43.491) (-8.3907, -43.4222) (-8.3375, -43.3533) (-8.2848, -43.2842) (-8.2323, -43.215) (-8.1803, -43.1456) (-8.1286, -43.076) (-8.0773, -43.0063) (-8.0264, -42.9365) (-7.9759, -42.8665) (-7.9257, -42.7963) (-7.8759, -42.726) (-7.8265, -42.6555) (-7.7775, -42.5849) (-7.7289, -42.5141) (-7.6808, -42.4432) (-7.633, -42.3721) (-7.5856, -42.3008) (-7.5386, -42.2294) (-7.4921, -42.1579) (-7.4459, -42.0861) (-7.4003, -42.0143) (-7.355, -41.9423) (-7.3102, -41.8701) (-7.2658, -41.7978) (-7.2218, -41.7253) (-7.1783, -41.6526) (-7.1353, -41.5798) (-7.0927, -41.5069) (-7.0506, -41.4338) (-7.009, -41.3605) (-6.9679, -41.2871) (-6.9272, -41.2135) (-6.8871, -41.1398) (-6.8475, -41.0659) (-6.8084, -40.9918) (-6.7697, -40.9176) (-6.7316, -40.8432) (-6.6941, -40.7687) (-6.6571, -40.694) (-6.6207, -40.6191) (-6.5849, -40.5441) (-6.5498, -40.4689) (-6.5152, -40.3935) (-6.4813, -40.3179) (-6.4479, -40.2422) (-6.4151, -40.1664) (-6.3829, -40.0904) (-6.3513, -40.0142) (-6.3206, -39.9378) (-6.2908, -39.8612) (-6.262, -39.7844) (-6.2343, -39.7073) (-6.2074, -39.63) (-6.1813, -39.5525) (-6.1556, -39.4749) (-6.1304, -39.3973) (-6.1059, -39.3195) (-6.0828, -39.2414) (-6.0618, -39.1629) (-6.0474, -39.0996) (-6.0382, -39.0518) (-6.0328, -39.0197) (-6.0303, -39.0037) knots -1 -1 -1 -1 -1 -1 -0.98571429 -0.97142857 -0.95714286 -0.94285714 -0.92857143 -0.91428571 -0.9 -0.88571429 -0.87142857 -0.85714286 -0.84285714 -0.82857143 -0.81428571 -0.8 -0.78571429 -0.77142857 -0.75714286 -0.74285714 -0.72857143 -0.71428571 -0.7 -0.68571429 -0.67142857 -0.65714286 -0.64285714 -0.62857143 -0.61428571 -0.6 -0.58571429 -0.57142857 -0.55714286 -0.54285714 -0.52857143 -0.51428571 -0.5 -0.48571429 -0.47142857 -0.45714286 -0.44285714 -0.42857143 -0.41428571 -0.4 -0.38571429 -0.37142857 -0.35714286 -0.34285714 -0.32857143 -0.31428571 -0.3 -0.28571429 -0.27142857 -0.25714286 -0.24285714 -0.22857143 -0.21428571 -0.2 -0.18571429 -0.17142857 -0.15714286 -0.14285714 -0.12857143 -0.11428571 -0.1 -0.08571429 -0.07142857 -0.05714286 -0.04285714 -0.02857143 -0.01428571 0 0 0 0 0 0
  line L13 (-6.0303, -39.0037) -> (-6.0102, -38.874)
  arc A27 (-4.8944, -38.0356) -> (-6.0102, -38.874) centre (-5.0221, -39.0274) ccw
  arc A28 (-4.8944, -38.0356) -> (-3.692, -38.1711) centre (0, 0) ccw
  arc A29 (-2.7907, -39.2367) -> (-3.692, -38.1711) centre (-3.7883, -39.1664) ccw
  line L14 (-2.7907, -39.2367) -> (-2.8, -39.3676)
  spline S14 degree 5 poles (-2.8, -39.3676) (-2.8011, -39.3839) (-2.803, -39.4163) (-2.8047, -39.4649) (-2.8047, -39.5299) (-2.8017, -39.6111) (-2.7966, -39.6923) (-2.79, -39.7736) (-2.7828, -39.855) (-2.775, -39.9363) (-2.7667, -40.0176) (-2.7577, -40.099) (-2.7478, -40.1803) (-2.7369, -40.2616) (-2.7249, -40.343) (-2.7119, -40.4243) (-2.6981, -40.5056) (-2.6836, -40.5868) (-2.6685, -40.6681) (-2.6528, -40.7493) (-2.6365, -40.8305) (-2.6196, -40.9117) (-2.6021, -40.9928) (-2.5839, -41.074) (-2.5651, -41.1551) (-2.5457, -41.2361) (-2.5256, -41.3171) (-2.505, -41.3981) (-2.4839, -41.4791) (-2.4622, -41.56) (-2.44, -41.6408) (-2.4173, -41.7216) (-2.3941, -41.8024) (-2.3703, -41.8832) (-2.346, -41.9638) (-2.3213, -42.0445) (-2.296, -42.1251) (-2.2702, -42.2056) (-2.244, -42.2861) (-2.2173, -42.3666) (-2.1901, -42.447) (-2.1624, -42.5273) (-2.1343, -42.6076) (-2.1058, -42.6878) (-2.0768, -42.768) (-2.0473, -42.8481) (-2.0174, -42.9282) (-1.9871, -43.0082) (-1.9563, -43.0881) (-1.9251, -43.168) (-1.8935, -43.2479) (-1.8614, -43.3276) (-1.829, -43.4073) (-1.7961, -43.4869) (-1.7628, -43.5665) (-1.7291, -43.646) (-1.695, -43.7254) (-1.6605, -43.8048) (-1.6256, -43.8841) (-1.5903, -43.9633) (-1.5546, -44.0425) (-1.5185, -44.1216) (-1.482, -44.2006) (-1.4452, -44.2795) (-1.4079, -44.3584) (-1.3703, -44.4372) (-1.3323, -44.5159) (-1.2939, -44.5946) (-1.2552, -44.6732) (-1.2161, -44.7516) (-1.1766, -44.8301) (-1.1447, -44.8927) (-1.1206, -44.9397) (-1.1045, -44.971) (-1.0964, -44.9866) knots 0 0 0 0 0 0 0.01428571 0.02857143 0.04285714 0.05714286 0.07142857 0.08571429 0.1 0.11428571 0.12857143 0.14285714 0.15714286 0.17142857 0.18571429 0.2 0.21428571 0.22857143 0.24285714 0.25714286 0.27142857 0.28571429 0.3 0.31428571 0.32857143 0.34285714 0.35714286 0.37142857 0.38571429 0.4 0.41428571 0.42857143 0.44285714 0.45714286 0.47142857 0.48571429 0.5 0.51428571 0.52857143 0.54285714 0.55714286 0.57142857 0.58571429 0.6 0.61428571 0.62857143 0.64285714 0.65714286 0.67142857 0.68571429 0.7 0.71428571 0.72857143 0.74285714 0.75714286 0.77142857 0.78571429 0.8 0.81428571 0.82857143 0.84285714 0.85714286 0.87142857 0.88571429 0.9 0.91428571 0.92857143 0.94285714 0.95714286 0.97142857 0.98571429 1 1 1 1 1 1
  arc A30 (-1.0964, -44.9866) -> (1.0964, -44.9866) centre (0, 0) ccw
  spline S15 degree 5 poles (1.0964, -44.9866) (1.1045, -44.971) (1.1206, -44.9397) (1.1447, -44.8927) (1.1766, -44.8301) (1.2161, -44.7516) (1.2552, -44.6732) (1.2939, -44.5946) (1.3323, -44.5159) (1.3703, -44.4372) (1.4079, -44.3584) (1.4452, -44.2795) (1.482, -44.2006) (1.5185, -44.1216) (1.5546, -44.0425) (1.5903, -43.9633) (1.6256, -43.8841) (1.6605, -43.8048) (1.695, -43.7254) (1.7291, -43.646) (1.7628, -43.5665) (1.7961, -43.4869) (1.829, -43.4073) (1.8614, -43.3276) (1.8935, -43.2479) (1.9251, -43.168) (1.9563, -43.0881) (1.9871, -43.0082) (2.0174, -42.9282) (2.0473, -42.8481) (2.0768, -42.768) (2.1058, -42.6878) (2.1343, -42.6076) (2.1624, -42.5273) (2.1901, -42.447) (2.2173, -42.3666) (2.244, -42.2861) (2.2702, -42.2056) (2.296, -42.1251) (2.3213, -42.0445) (2.346, -41.9638) (2.3703, -41.8832) (2.3941, -41.8024) (2.4173, -41.7216) (2.44, -41.6408) (2.4622, -41.56) (2.4839, -41.4791) (2.505, -41.3981) (2.5256, -41.3171) (2.5457, -41.2361) (2.5651, -41.1551) (2.5839, -41.074) (2.6021, -40.9928) (2.6196, -40.9117) (2.6365, -40.8305) (2.6528, -40.7493) (2.6685, -40.6681) (2.6836, -40.5868) (2.6981, -40.5056) (2.7119, -40.4243) (2.7249, -40.343) (2.7369, -40.2616) (2.7478, -40.1803) (2.7577, -40.099) (2.7667, -40.0176) (2.775, -39.9363) (2.7828, -39.855) (2.79, -39.7736) (2.7966, -39.6923) (2.8017, -39.6111) (2.8047, -39.5299) (2.8047, -39.4649) (2.803, -39.4163) (2.8011, -39.3839) (2.8, -39.3676) knots -1 -1 -1 -1 -1 -1 -0.98571429 -0.97142857 -0.95714286 -0.94285714 -0.92857143 -0.91428571 -0.9 -0.88571429 -0.87142857 -0.85714286 -0.84285714 -0.82857143 -0.81428571 -0.8 -0.78571429 -0.77142857 -0.75714286 -0.74285714 -0.72857143 -0.71428571 -0.7 -0.68571429 -0.67142857 -0.65714286 -0.64285714 -0.62857143 -0.61428571 -0.6 -0.58571429 -0.57142857 -0.55714286 -0.54285714 -0.52857143 -0.51428571 -0.5 -0.48571429 -0.47142857 -0.45714286 -0.44285714 -0.42857143 -0.41428571 -0.4 -0.38571429 -0.37142857 -0.35714286 -0.34285714 -0.32857143 -0.31428571 -0.3 -0.28571429 -0.27142857 -0.25714286 -0.24285714 -0.22857143 -0.21428571 -0.2 -0.18571429 -0.17142857 -0.15714286 -0.14285714 -0.12857143 -0.11428571 -0.1 -0.08571429 -0.07142857 -0.05714286 -0.04285714 -0.02857143 -0.01428571 0 0 0 0 0 0
  line L15 (2.8, -39.3676) -> (2.7907, -39.2367)
  arc A31 (3.692, -38.1711) -> (2.7907, -39.2367) centre (3.7883, -39.1664) ccw
  arc A32 (3.692, -38.1711) -> (4.8944, -38.0356) centre (0, 0) ccw
  arc A33 (6.0102, -38.874) -> (4.8944, -38.0356) centre (5.0221, -39.0274) ccw
  line L16 (6.0102, -38.874) -> (6.0303, -39.0037)
  spline S16 degree 5 poles (6.0303, -39.0037) (6.0328, -39.0197) (6.0382, -39.0518) (6.0474, -39.0996) (6.0618, -39.1629) (6.0828, -39.2414) (6.1059, -39.3195) (6.1304, -39.3973) (6.1556, -39.4749) (6.1813, -39.5525) (6.2074, -39.63) (6.2343, -39.7073) (6.262, -39.7844) (6.2908, -39.8612) (6.3206, -39.9378) (6.3513, -40.0142) (6.3829, -40.0904) (6.4151, -40.1664) (6.4479, -40.2422) (6.4813, -40.3179) (6.5152, -40.3935) (6.5498, -40.4689) (6.5849, -40.5441) (6.6207, -40.6191) (6.6571, -40.694) (6.6941, -40.7687) (6.7316, -40.8432) (6.7697, -40.9176) (6.8084, -40.9918) (6.8475, -41.0659) (6.8871, -41.1398) (6.9272, -41.2135) (6.9679, -41.2871) (7.009, -41.3605) (7.0506, -41.4338) (7.0927, -41.5069) (7.1353, -41.5798) (7.1783, -41.6526) (7.2218, -41.7253) (7.2658, -41.7978) (7.3102, -41.8701) (7.355, -41.9423) (7.4003, -42.0143) (7.4459, -42.0861) (7.4921, -42.1579) (7.5386, -42.2294) (7.5856, -42.3008) (7.633, -42.3721) (7.6808, -42.4432) (7.7289, -42.5141) (7.7775, -42.5849) (7.8265, -42.6555) (7.8759, -42.726) (7.9257, -42.7963) (7.9759, -42.8665) (8.0264, -42.9365) (8.0773, -43.0063) (8.1286, -43.076) (8.1803, -43.1456) (8.2323, -43.215) (8.2848, -43.2842) (8.3375, -43.3533) (8.3907, -43.4222) (8.4442, -43.491) (8.498, -43.5596) (8.5523, -43.628) (8.6068, -43.6963) (8.6617, -43.7644) (8.717, -43.8324) (8.7726, -43.9002) (8.8285, -43.9679) (8.8736, -44.0219) (8.9075, -44.0623) (8.9302, -44.0893) (8.9415, -44.1027) knots 0 0 0 0 0 0 0.01428571 0.02857143 0.04285714 0.05714286 0.07142857 0.08571429 0.1 0.11428571 0.12857143 0.14285714 0.15714286 0.17142857 0.18571429 0.2 0.21428571 0.22857143 0.24285714 0.25714286 0.27142857 0.28571429 0.3 0.31428571 0.32857143 0.34285714 0.35714286 0.37142857 0.38571429 0.4 0.41428571 0.42857143 0.44285714 0.45714286 0.47142857 0.48571429 0.5 0.51428571 0.52857143 0.54285714 0.55714286 0.57142857 0.58571429 0.6 0.61428571 0.62857143 0.64285714 0.65714286 0.67142857 0.68571429 0.7 0.71428571 0.72857143 0.74285714 0.75714286 0.77142857 0.78571429 0.8 0.81428571 0.82857143 0.84285714 0.85714286 0.87142857 0.88571429 0.9 0.91428571 0.92857143 0.94285714 0.95714286 0.97142857 0.98571429 1 1 1 1 1 1
  arc A34 (8.9415, -44.1027) -> (11.0794, -43.6148) centre (0, 0) ccw
  spline S17 degree 5 poles (11.0794, -43.6148) (11.0838, -43.5977) (11.0926, -43.5636) (11.1056, -43.5125) (11.1227, -43.4443) (11.1438, -43.359) (11.1644, -43.2738) (11.1847, -43.1886) (11.2046, -43.1034) (11.2242, -43.0182) (11.2433, -42.933) (11.2621, -42.8478) (11.2804, -42.7626) (11.2984, -42.6775) (11.316, -42.5923) (11.3332, -42.5072) (11.35, -42.4221) (11.3664, -42.337) (11.3823, -42.252) (11.3979, -42.167) (11.4131, -42.0819) (11.4278, -41.997) (11.4422, -41.912) (11.4561, -41.8271) (11.4696, -41.7422) (11.4826, -41.6573) (11.4953, -41.5725) (11.5075, -41.4877) (11.5193, -41.403) (11.5306, -41.3183) (11.5415, -41.2336) (11.5519, -41.149) (11.5619, -41.0644) (11.5715, -40.9799) (11.5805, -40.8954) (11.5891, -40.811) (11.5973, -40.7266) (11.6049, -40.6423) (11.6121, -40.558) (11.6188, -40.4738) (11.6251, -40.3897) (11.6308, -40.3056) (11.636, -40.2216) (11.6406, -40.1377) (11.6448, -40.0538) (11.6484, -39.9701) (11.6516, -39.8864) (11.6542, -39.8028) (11.6562, -39.7192) (11.6577, -39.6358) (11.6587, -39.5524) (11.659, -39.4692) (11.6586, -39.3861) (11.6577, -39.303) (11.656, -39.2201) (11.6538, -39.1373) (11.6511, -39.0547) (11.6477, -38.9721) (11.6438, -38.8896) (11.6392, -38.8073) (11.6337, -38.7251) (11.6273, -38.6432) (11.6199, -38.5615) (11.6114, -38.48) (11.6021, -38.3987) (11.5921, -38.3175) (11.5816, -38.2365) (11.5706, -38.1556) (11.5588, -38.0749) (11.5458, -37.9945) (11.5306, -37.9147) (11.5162, -37.8514) (11.5037, -37.8043) (11.4946, -37.7731) (11.4899, -37.7576) knots -1 -1 -1 -1 -1 -1 -0.98571429 -0.97142857 -0.95714286 -0.94285714 -0.92857143 -0.91428571 -0.9 -0.88571429 -0.87142857 -0.85714286 -0.84285714 -0.82857143 -0.81428571 -0.8 -0.78571429 -0.77142857 -0.75714286 -0.74285714 -0.72857143 -0.71428571 -0.7 -0.68571429 -0.67142857 -0.65714286 -0.64285714 -0.62857143 -0.61428571 -0.6 -0.58571429 -0.57142857 -0.55714286 -0.54285714 -0.52857143 -0.51428571 -0.5 -0.48571429 -0.47142857 -0.45714286 -0.44285714 -0.42857143 -0.41428571 -0.4 -0.38571429 -0.37142857 -0.35714286 -0.34285714 -0.32857143 -0.31428571 -0.3 -0.28571429 -0.27142857 -0.25714286 -0.24285714 -0.22857143 -0.21428571 -0.2 -0.18571429 -0.17142857 -0.15714286 -0.14285714 -0.12857143 -0.11428571 -0.1 -0.08571429 -0.07142857 -0.05714286 -0.04285714 -0.02857143 -0.01428571 0 0 0 0 0 0
  line L17 (11.4899, -37.7576) -> (11.4518, -37.632)
  arc A35 (12.0933, -36.3925) -> (11.4518, -37.632) centre (12.4086, -37.3415) ccw
  arc A36 (12.0933, -36.3925) -> (13.2354, -35.9928) centre (0, 0) ccw
  arc A37 (14.5098, -36.5619) -> (13.2354, -35.9928) centre (13.5806, -36.9314) ccw
  line L18 (14.5098, -36.5619) -> (14.5583, -36.6839)
  spline S18 degree 5 poles (14.5583, -36.6839) (14.5643, -36.699) (14.5767, -36.729) (14.5962, -36.7736) (14.6244, -36.8321) (14.6623, -36.904) (14.7022, -36.975) (14.7434, -37.0454) (14.7852, -37.1155) (14.8275, -37.1854) (14.8703, -37.2551) (14.9137, -37.3245) (14.9579, -37.3935) (15.003, -37.462) (15.0491, -37.5301) (15.0961, -37.5977) (15.1438, -37.6649) (15.1921, -37.7319) (15.241, -37.7985) (15.2904, -37.8649) (15.3403, -37.931) (15.3907, -37.9968) (15.4417, -38.0623) (15.4933, -38.1275) (15.5454, -38.1924) (15.5981, -38.257) (15.6513, -38.3213) (15.705, -38.3853) (15.7592, -38.449) (15.8138, -38.5125) (15.8689, -38.5758) (15.9244, -38.6387) (15.9804, -38.7014) (16.0368, -38.7639) (16.0937, -38.826) (16.151, -38.8879) (16.2088, -38.9496) (16.2669, -39.011) (16.3255, -39.0721) (16.3845, -39.133) (16.4438, -39.1937) (16.5036, -39.254) (16.5638, -39.3142) (16.6243, -39.3741) (16.6852, -39.4337) (16.7465, -39.4931) (16.8082, -39.5523) (16.8703, -39.6112) (16.9327, -39.6699) (16.9954, -39.7283) (17.0586, -39.7865) (17.122, -39.8445) (17.1859, -39.9022) (17.25, -39.9597) (17.3146, -40.0169) (17.3794, -40.0739) (17.4446, -40.1307) (17.5101, -40.1872) (17.576, -40.2435) (17.6422, -40.2996) (17.7087, -40.3554) (17.7755, -40.411) (17.8427, -40.4664) (17.9101, -40.5215) (17.9779, -40.5764) (18.046, -40.6311) (18.1144, -40.6855) (18.1831, -40.7398) (18.2521, -40.7937) (18.3214, -40.8475) (18.391, -40.901) (18.4469, -40.9436) (18.4889, -40.9755) (18.5171, -40.9967) (18.5311, -41.0073) knots 0 0 0 0 0 0 0.01428571 0.02857143 0.04285714 0.05714286 0.07142857 0.08571429 0.1 0.11428571 0.12857143 0.14285714 0.15714286 0.17142857 0.18571429 0.2 0.21428571 0.22857143 0.24285714 0.25714286 0.27142857 0.28571429 0.3 0.31428571 0.32857143 0.34285714 0.35714286 0.37142857 0.38571429 0.4 0.41428571 0.42857143 0.44285714 0.45714286 0.47142857 0.48571429 0.5 0.51428571 0.52857143 0.54285714 0.55714286 0.57142857 0.58571429 0.6 0.61428571 0.62857143 0.64285714 0.65714286 0.67142857 0.68571429 0.7 0.71428571 0.72857143 0.74285714 0.75714286 0.77142857 0.78571429 0.8 0.81428571 0.82857143 0.84285714 0.85714286 0.87142857 0.88571429 0.9 0.91428571 0.92857143 0.94285714 0.95714286 0.97142857 0.98571429 1 1 1 1 1 1
  arc A38 (18.5311, -41.0073) -> (20.5068, -40.0558) centre (0, 0) ccw